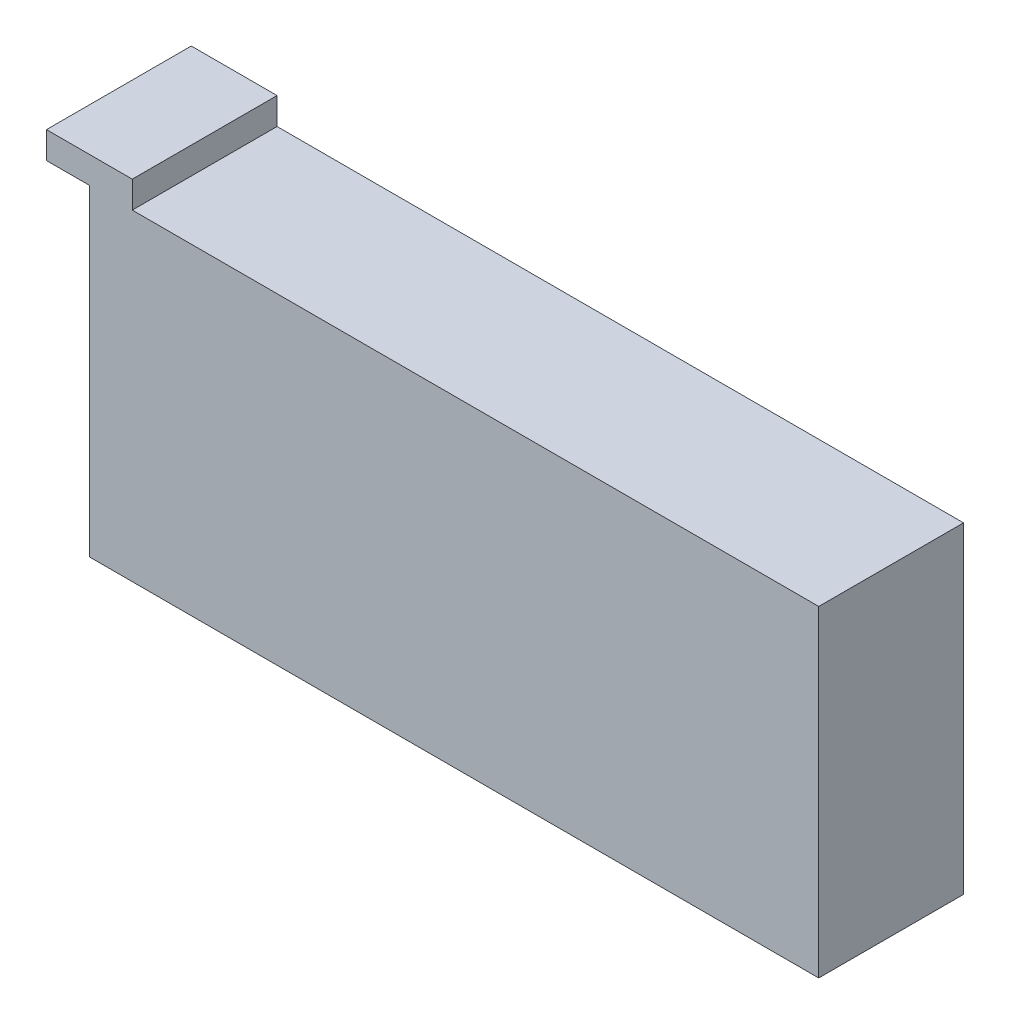
# Autodesk Inventor part: nVision lipo battery
Saved by Autodesk Inventor 2020 (Build 240168000, 168)
## iProperties
Created: 2021-02-21
Part Number: nVision lipo battery
Material: Типовые
Document SubType Name: Modeling
Designer: Антон
Density: 1 g/cm^3
Appearance: По умолчанию
Author: Антон
Autodesk Inventor part; units mm, degrees
ref_plane "YZ Plane" through (0, 0, 0) normal (1, 0, 0) x (0, 1, 0)
ref_plane "XZ Plane" through (0, 0, 0) normal (0, 1, 0) x (-1, 0, 0)
ref_plane "XY Plane" through (0, 0, 0) normal (0, 0, 1) x (1, 0, 0)
sketch "Эскиз1" plane through (0, 0, 0) normal (0, 0, 1) x (1, 0, 0)
  line L0 (0, 0) -> (68, 0)
  line L1 (68, 0) -> (68, 30)
  line L2 (68, 30) -> (0, 30)
  line L3 (0, 30) -> (0, 0)
  line L4 (0, 30) -> (4, 30)
  line L5 (4, 30) -> (-4, 30)
  line L6 (-4, 30) -> (-4, 32.5)
  line L7 (-4, 32.5) -> (4, 32.5)
  line L8 (4, 32.5) -> (4, 30)
  dimension "d0" = 68
  dimension "d1" = 30
  dimension "d4" = 4
  dimension "d5" = 8
  dimension "d6" = 2.5
  constraints: 18 end point, 4 parallel, 2 horizontal, 2 perpendicular, 1 point on line
  measures "d0" distance of L2.end L1.end
  measures "d1" distance of L1.end L0.end
  measures "d4" distance of L2.end L4.end
  measures "d5" distance of L6.end L7.end
  measures "d6" distance of L5.end L6.end
extrude "Выдавливание1" add sketch "Эскиз1" along normal blind 13.5
